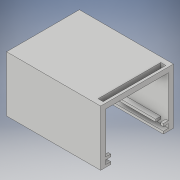
# Autodesk Inventor part: bens capstone
Saved by Autodesk Inventor 2017 (Build 210142000, 142)
## iProperties
Created: 2021-04-14
Part Number: bens capstone
Material: Generic
Document SubType Name: Modeling
Designer: jenna
Density: 1 g/cm^3
Appearance: Default
Author: jenna
Autodesk Inventor part; units mm, degrees
ref_plane "YZ Plane" through (0, 0, 0) normal (1, 0, 0) x (0, 1, 0)
ref_plane "XZ Plane" through (0, 0, 0) normal (0, 1, 0) x (-1, 0, 0)
ref_plane "XY Plane" through (0, 0, 0) normal (0, 0, 1) x (1, 0, 0)
sketch "Sketch1" plane through (0, 0, 0) normal (1, 0, 0) x (0, 1, 0)
  point P0 (0, 0)
sketch "Sketch2" plane through (0, 0, 0) normal (1, 0, 0) x (0, 1, 0)
  line L0 (22.3119, 47.1251) -> (-47.5381, 47.1251)
  line L1 (-47.5381, 47.1251) -> (-47.5381, -44.3149)
  line L2 (-47.5381, -44.3149) -> (22.3119, -44.3149)
  line L3 (22.3119, -44.3149) -> (22.3119, 47.1251)
  point P0 (0, 0)
  dimension "d0" = 91.44
  dimension "d1" = 69.85
  constraints: 8 end point, 2 parallel, 1 horizontal, 1 perpendicular
  measures "d0" distance of L2.end L0.start
  measures "d1" distance of L1.end L2.end
extrude "Extrusion1" add sketch "Sketch2" along normal blind 6.35
sketch "Sketch3" plane through (6.35, 0, 0) normal (1, 0, 0) x (0, 0, -1)
  line L0 (-47.1251, 22.3119) -> (-47.1251, -47.5381) projected
  line L1 (-47.1251, -47.5381) -> (-47.1251, 22.3119)
  line L2 (44.3149, -47.5381) -> (44.3149, 22.3119) projected
  line L3 (-47.1251, 22.3119) -> (44.3149, 22.3119)
  line L4 (44.3149, 22.3119) -> (44.3149, -47.5381)
  line L5 (-47.1251, -47.5381) -> (-40.7751, -47.5381)
  line L6 (-47.1251, -47.5381) -> (44.3149, -47.5381) projected
  line L7 (37.9649, -47.5381) -> (44.3149, -47.5381)
  line L8 (-40.7751, -47.5381) -> (-34.4251, -47.5381)
  line L9 (37.9649, -47.5381) -> (31.6149, -47.5381)
  line L10 (31.6149, -47.5381) -> (31.6149, -44.3631)
  line L11 (31.6149, -44.3631) -> (37.9649, -44.3631)
  line L12 (-34.4251, -47.5381) -> (-34.4251, -44.3631)
  line L13 (-34.4251, -44.3631) -> (-40.7751, -44.3631)
  line L14 (-40.7751, 15.9619) -> (37.9649, 15.9619)
  line L15 (-40.7751, -33.5681) -> (-40.7751, 15.9619)
  line L16 (37.9649, 15.9619) -> (37.9649, -33.5681)
  line L17 (-40.7751, -44.3631) -> (-40.7751, -39.2831)
  line L18 (-40.7751, -39.2831) -> (-34.4251, -39.2831)
  line L19 (-34.4251, -39.2831) -> (-34.4251, -36.1081)
  line L20 (-34.4251, -36.1081) -> (-40.7751, -36.1081)
  line L21 (-40.7751, -36.1081) -> (-40.7751, -33.5681)
  line L22 (37.9649, -44.3631) -> (37.9649, -39.2831)
  line L23 (37.9649, -39.2831) -> (31.6149, -39.2831)
  line L24 (31.6149, -39.2831) -> (31.6149, -36.1081)
  line L25 (31.6149, -36.1081) -> (37.9649, -36.1081)
  line L26 (37.9649, -36.1081) -> (37.9649, -33.5681)
  point P0 (0, 0)
  dimension "d7" = 78.74
  dimension "d10" = 6.35
  dimension "d11" = 3.175
  dimension "d25" = 3.175
  dimension "d26" = 5.08
  dimension "d27" = 5.08
  dimension "d28" = 3.175
  dimension "d29" = 3.175
  dimension "d30" = 6.35
  dimension "d31" = 66.04
  constraints: 48 end point, 14 perpendicular, 7 point on line, 3 collinear, 2 vertical
  measures "d7" distance of L14.start L14.end
  measures "d10" distance of L7.start L9.end
  measures "d11" distance of L9.end L10.end
  measures "d25" distance of L18.end L19.end
  measures "d26" distance of L11.end L22.end
  measures "d27" distance of L13.end L17.end
  measures "d28" distance of L8.end L12.end
  measures "d29" distance of L23.end L24.end
  measures "d30" distance of L5.end L8.end
  measures "d31" distance between parallel lines of L24 L19
extrude "Extrusion2" add sketch "Sketch3" along normal blind 111.76 contours L3 L2 L6 L10 L11 L22 L23 L24 L25 L26 L16 L14 L15 L21 L20 L19 L18 L17 L13 L12 L5 L0
sketch "Sketch4" plane through (0, 22.3119, 47.1251) normal (0, 1, 0) x (1, 0, 0)
  line L0 (114.935, 6.35) -> (114.935, 85.09)
  line L1 (114.935, 6.35) -> (108.585, 6.35)
  line L2 (108.585, 6.35) -> (108.585, 85.09)
  line L3 (114.935, 85.09) -> (108.585, 85.09)
  point P0 (0, 47.1251)
  constraints: 8 end point, 2 perpendicular
extrude "Extrusion3" cut sketch "Sketch4" against normal blind 63.5
body "Solid1"
